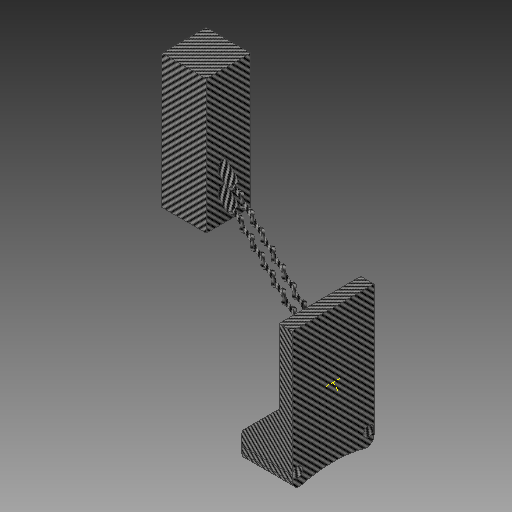
# Autodesk Inventor part: lower clamp
Saved by Autodesk Inventor 2018 (Build 220112000, 112)
## iProperties
Created: 2021-03-10
Part Number: lower clamp
Material: CFRP
Document SubType Name: Modeling
Designer: Hp
Density: 1.43 g/cm^3
Appearance: Carbon Fiber
Author: Hp
Autodesk Inventor part; units mm, degrees
sketch "Sketch1" plane through (0, 0, 0) normal (0, 1, 0) x (-1, 0, 0)
  line L0 (0, 0) -> (34, 0)
  line L1 (34, 0) -> (34, -55)
  line L2 (34, -55) -> (0, -55)
  line L3 (0, -55) -> (0, 0)
  dimension "d0" = 34
  dimension "d1" = 55
  dimension "d2" = 90
  dimension "d3" = 34
  dimension "d4" = 90
  constraints: 8 end point, 2 perpendicular, 1 horizontal
  measures "d0" distance of L0.start L0.end
  measures "d1" distance of L0.end L1.end
  measures "d2" angle of L0 L1
  measures "d3" distance of L1.end L2.end
  measures "d4" angle of L1 L2
extrude "Extrusion1" add sketch "Sketch1" along normal blind 9
sketch "Sketch2" plane through (0, 0, 0) normal (1, 0, 0) x (0, 0, -1)
  line L0 (55, 0) -> (0, 0) projected
  arc A0 (7, 0) -> (0, 0) centre (3.5, 0) ccw
  arc A1 (55, 0) -> (48, 0) centre (51.5, 0) ccw
  dimension "d7" = 7
  dimension "d8" = 7
  constraints: 4 point on circle, 4 point on line, 2 centre point, 2 end point
  measures "d7" diameter of A0
  measures "d8" diameter of A1
extrude "Extrusion2" cut sketch "Sketch2" against normal blind 1000
sketch "Sketch3" plane through (-34, 9, 0) normal (0, 0, 1) x (1, 0, 0)
  line L0 (0, 0) -> (34, 0) projected
  line L1 (34, 0) -> (34, 50)
  line L2 (0, 0) -> (25, 25)
  line L3 (0, 0) -> (50.7113, 0) construction
  line L4 (25, 25) -> (25, 50) construction
  line L5 (25, 25) -> (25, 50)
  line L6 (34, 50) -> (25, 50)
  point P0 (34, -9)
  dimension "d11" = 50
  dimension "d12" = 45
  dimension "d13" = 9
  constraints: 12 end point, 2 vertical, 1 collinear, 1 horizontal, 1 perpendicular
  measures "d11" distance of L0.end L1.end
  measures "d12" angle of L3 L2
  measures "d13" distance of L1.end L4.end
extrude "Extrusion3" add sketch "Sketch3" against normal blind 55
sketch "Sketch4" plane through (0, 0, 0) normal (0, -1, 0) x (1, 0, 0)
  line L0 (-34, -55) -> (-9, -55) projected
  line L1 (-9, 0) -> (-34, 0) projected
  circle A0 centre (-17, -27.5) radius 3.5
  point P0 (0, 0)
  dimension "d16" = 7
  constraints: 1 centre point
  measures "d16" diameter of A0
extrude "Extrusion4" add sketch "Sketch4" against normal blind 30 and the other way blind 10
sketch "Sketch5" plane through (-9, 59, 0) normal (0, 1, 0) x (1, 0, 0)
  line L0 (0, 0) -> (0, 55) projected
  line L1 (0, 55) -> (9, 55) projected
  line L2 (0, 0) -> (9, 0)
  line L3 (9, 0) -> (9, 55)
  line L4 (9, 55) -> (0, 55)
  line L5 (0, 55) -> (0, 0)
  constraints: 8 end point, 2 parallel, 1 horizontal, 1 perpendicular
extrude "Extrusion5" add sketch "Sketch5" along normal blind 5
sketch "Sketch7" plane through (0, 0, -7) normal (1, 0, 0) x (0, 0, -1)
  circle A0 centre (20.5, 44) radius 3.5 projected
  circle A1 centre (20.5, 44) radius 3.5
  circle A2 centre (20.5, 54) radius 3.5 projected
  circle A3 centre (20.5, 54) radius 3.5
  point P0 (-7, 0)
  constraints: 2 centre point, 2 coincident
extrude "Extrusion7" add sketch "Sketch7" against normal blind 9
sketch "Sketch15" plane through (-9, 64, 0) normal (0, 1, 0) x (1, 0, 0)
  line L0 (-25, 55) -> (9, 55) projected
  line L1 (0, 0) -> (9, 0)
  line L2 (9, 0) -> (9, 55)
  line L3 (9, 55) -> (0, 55)
  line L4 (0, 55) -> (0, 0)
  constraints: 8 end point, 2 parallel, 1 horizontal, 1 perpendicular
extrude "Extrusion9" add sketch "Sketch15" along normal blind 20
ref_plane "Work Plane4" through (-9, 84, -55) normal (-0.7071068, 0.7071068, 0) x (0, 0, 1)
sketch "Sketch17" plane through (-9, 84, -55) normal (-0.7071068, 0.7071068, 0) x (0, 0, 1)
  line L0 (0, 0) -> (55, 0) construction
  line L1 (27.5, 0) -> (27.5, -14.414) construction
  circle A0 centre (27.5, -14.414) radius 3.5 construction
  circle A1 centre (27.5, -14.414) radius 3.5
  line L2 (27.5, -14.414) -> (27.5, -24.414) construction
  circle A2 centre (27.5, -24.414) radius 3.5 construction
  circle A3 centre (27.5, -24.414) radius 3.5
  point P0 (55, -53.033)
  dimension "d49" = 14.414
  dimension "d50" = 7
  dimension "d51" = 10
  dimension "d52" = 7
  dimension "d53" = 7
  constraints: 4 centre point, 4 coincident, 4 end point, 1 concentric, 1 midpoint, 1 point on line, 1 vertical
  measures "d49" distance of L1.start L1.end
  measures "d50" diameter of A0
  measures "d51" distance of L2.start L2.end
  measures "d52" diameter of A2
  measures "d53" diameter of A3
extrude "Extrusion11" cut sketch "Sketch17" against normal blind 200
sketch "Sketch18" plane through (0, 40.4734, -27.5) normal (0.7071068, 0.7071068, 0) x (0, 0, -1)
  point P0 (0, 0)
sketch "Sketch19" plane through (0, 40.4734, -27.5) normal (-0.7071068, 0.7071068, 0) x (0.7071068, 0.7071068, 0)
  circle A0 centre (0, 0) radius 3.5
  circle A1 centre (0, 0) radius 2.5
  dimension "d68" = 5
  constraints: 2 centre point, 2 coincident
  measures "d68" diameter of A1
extrude "Extrusion12" add sketch "Sketch19" along normal blind 20 and the other way blind 10
sketch "Sketch21" plane through (0, 40.4734, -27.5) normal (-0.7071068, 0.7071068, 0) x (0.7071068, 0.7071068, 0)
  circle A0 centre (0, 0) radius 2.5
  constraints: 1 centre point, 1 coincident
extrude "Extrusion13" add sketch "Sketch21" along normal blind 18 and the other way blind 10
sketch "Sketch23" plane through (-12.7279, 53.2013, -27.5) normal (-0.7071068, 0.7071068, 0) x (-0.7071068, -0.7071068, 0)
  circle A0 centre (-1.5, 0) radius 1
  point P0 (28.619, 27.5)
  constraints: 1 centre point
coil "Coil1" sketch "Sketch23" operation add axis through (7.0711, 33.4023, -27.5) along (-0.7071068, 0.7071068, 0) pitch 10 turns 8 hand right
sketch "Sketch24" plane through (0, 54.6155, -27.5) normal (-0.7071068, 0.7071068, 0) x (-0.7071068, -0.7071068, 0)
  circle A0 centre (0, 0) radius 3.5
  circle A1 centre (0, 0) radius 2.5
  dimension "d91" = 5
  constraints: 2 centre point, 2 coincident
  measures "d91" diameter of A1
extrude "Extrusion14" add sketch "Sketch24" along normal blind 20 and the other way blind 10
sketch "Sketch25" plane through (0, 54.6155, -27.5) normal (0, 0, 1) x (-0.7071068, 0.7071068, 0)
  point P0 (0, 0)
sketch "Sketch26" plane through (0, 54.6155, -27.5) normal (-0.7071068, 0.7071068, 0) x (-0.7071068, -0.7071068, 0)
  circle A0 centre (0, 0) radius 2.5
  constraints: 1 centre point, 1 coincident
extrude "Extrusion15" add sketch "Sketch26" along normal blind 18 and the other way blind 10
sketch "Sketch27" plane through (-12.7279, 67.3434, -27.5) normal (-0.7071068, 0.7071068, 0) x (-0.7071068, -0.7071068, 0)
  point P0 (38.619, 27.5)
sketch "Sketch28" plane through (-12.7279, 67.3434, -27.5) normal (-0.7071068, 0.7071068, 0) x (-0.7071068, -0.7071068, 0)
  circle A0 centre (-1.5, 0) radius 1
  point P0 (38.619, 27.5)
  dimension "d96" = 2
  constraints: 1 centre point
  measures "d96" diameter of A0
coil "Coil2" sketch "Sketch28" operation add axis through (7.0711, 47.5445, -27.5) along (-0.7071068, 0.7071068, 0) pitch 10 turns 8 hand right
ref_plane "Work Plane5" through (-70.7107, 111.1841, -27.5) normal (-0.7071068, 0.7071068, 0) x (-0.7071068, -0.7071068, 0)
sketch "Sketch29" plane through (-70.7107, 111.1841, -27.5) normal (-0.7071068, 0.7071068, 0) x (-0.7071068, -0.7071068, 0)
  circle A0 centre (0, 0) radius 2.5
  circle A1 centre (0, 0) radius 3.5
  point P0 (28.619, 27.5)
  point P1 (-0.7725, -2.3776)
  constraints: 2 coincident, 1 centre point, 3 other
extrude "Extrusion16" add sketch "Sketch29" along normal blind 50 and the other way blind 5 contours A0 | A1
ref_plane "Work Plane6" through (-70.7107, 125.3262, -27.5) normal (-0.7071068, 0.7071068, 0) x (-0.7071068, -0.7071068, 0)
sketch "Sketch30" plane through (-70.7107, 125.3262, -27.5) normal (-0.7071068, 0.7071068, 0) x (-0.7071068, -0.7071068, 0)
  circle A0 centre (0, 0) radius 3.5 projected
  circle A1 centre (0, 0) radius 3.5
  point P0 (38.619, 27.5)
  constraints: 1 centre point, 1 coincident
extrude "Extrusion17" add sketch "Sketch30" along normal blind 50 and the other way blind 5
ref_plane "Work Plane7" through (-89, 34, -55) normal (-1, 0, 0) x (0, 0, 1)
sketch "Sketch31" plane through (-89, 34, -55) normal (-1, 0, 0) x (0, 0, 1)
  line L0 (9, 62.2361) -> (39, 62.2361)
  line L1 (39, 62.2361) -> (39, 152.2361)
  line L2 (39, 152.2361) -> (9, 152.2361)
  line L3 (9, 152.2361) -> (9, 62.2361)
  line L4 (24, 87.7907) -> (24, 126.6815) projected
  line L5 (9, 62.2361) -> (39, 152.2361) construction
  line L6 (39, 62.2361) -> (9, 152.2361) construction
  point P0 (55, -34)
  point P1 (24, 107.2361)
  dimension "d122" = 30
  dimension "d123" = 90
  constraints: 12 end point, 3 midpoint, 2 parallel, 1 horizontal, 1 perpendicular
  measures "d122" distance of L2.end L1.end
  measures "d123" distance of L1.end L0.end
extrude "Extrusion18" add sketch "Sketch31" against normal blind 15 and the other way blind 15
sketch "Sketch32" plane through (0, 0, 0) normal (0, -1, 0) x (1, 0, 0)
  line L0 (-34, -55) -> (0, -55)
  line L1 (0, -55) -> (0, 0)
  line L2 (0, 0) -> (-34, 0)
  line L3 (-34, 0) -> (-34, -55)
  circle A0 centre (-17, -27.5) radius 3.5 projected
  line L4 (-34, -55) -> (0, 0) construction
  line L5 (0, -55) -> (-34, 0) construction
  constraints: 12 end point, 2 midpoint, 2 parallel, 1 horizontal, 1 perpendicular
extrude "Extrusion19" add sketch "Sketch32" along normal blind 9
mirror "Mirror1" about plane through (-17, 0, -27.5) normal (0, 1, 0) of "Extrusion2"
sketch "Sketch33" plane through (0, 84, 0) normal (1, 0, 0) x (0, 0, -1)
  line L0 (55, -93) -> (0, -93) projected
  line L1 (55, 0) -> (0, 0)
  line L2 (0, 0) -> (0, -93)
  line L3 (0, -93) -> (55, -93)
  line L4 (55, -93) -> (55, 0)
  point P0 (0, -84)
  constraints: 8 end point, 2 parallel, 1 horizontal, 1 perpendicular
extrude "Extrusion20" cut sketch "Sketch33" along normal blind 900
sketch "Sketch34" plane through (-104, 34, -55) normal (-1, 0, 0) x (0, 0, 1)
  line L0 (39, 152.2361) -> (9, 152.2361) projected
  line L1 (39, 62.2361) -> (39, 152.2361) projected
  line L2 (9, 152.2361) -> (39, 152.2361)
  line L3 (39, 152.2361) -> (39, 62.2361)
  line L4 (39, 62.2361) -> (9, 62.2361)
  line L5 (9, 62.2361) -> (9, 152.2361)
  point P0 (55, -34)
  constraints: 8 end point, 2 parallel, 1 horizontal, 1 perpendicular
extrude "Extrusion21" cut sketch "Sketch34" along normal blind 900
sketch "Sketch36" plane through (-67.1751, 121.7907, -27.5) normal (0.7071068, -0.7071068, 0) x (-0.7071068, -0.7071068, 0)
  circle A0 centre (0, 0) radius 1
  point P0 (38.619, -27.5)
  dimension "d142" = 2
  constraints: 1 centre point
  measures "d142" diameter of A0
extrude "Extrusion22" add sketch "Sketch36" along normal blind 90
sketch "Sketch37" plane through (-67.1751, 107.6485, -27.5) normal (0.7071068, -0.7071068, 0) x (-0.7071068, -0.7071068, 0)
  circle A0 centre (0, 0) radius 1
  point P0 (28.619, -27.5)
  dimension "d145" = 2
  constraints: 1 centre point
  measures "d145" diameter of A0
extrude "Extrusion23" add sketch "Sketch37" along normal blind 90
fillet "Fillet1" radius 5 1 edges at (-34, 9, -27.5)
fillet "Fillet2" radius 5 2 edges at (-17, -9, -55) (-17, -9, 0)
sketch "Sketch39" plane through (-34, 0, -3.5) normal (-1, 0, 0) x (0, 0, 1)
  line L0 (-1.5, -9) -> (-46.5, -9) projected
  arc A0 (-51.5, -4) -> (-46.5, -9) centre (-46.5, -4) ccw projected
  arc A1 (-1.5, -9) -> (-46.5, -9) centre (-24, -87.6764) ccw
  line L1 (-1.5, -9) -> (-46.5, -9)
  point P0 (3.5, 0)
  constraints: 2 end point, 2 point on circle, 1 centre point, 1 collinear
extrude "Extrusion24" cut sketch "Sketch39" against normal blind 90
ref_plane "Work Plane10" through (-10.4142, 35.4142, -55) normal (-0.7071068, 0.7071068, 0) x (-0.7071068, -0.7071068, 0)
sketch "Sketch44" plane through (-10.4142, 35.4142, -55) normal (-0.7071068, 0.7071068, 0) x (-0.7071068, -0.7071068, 0)
  ellipse E0 centre (11.3137, 27.5) end of major axis (16.2635, 27.5) minor radius 3.5 projected
  circle A0 centre (11.3137, 27.5) radius 5
  point P0 (17.6777, 55)
  dimension "d163" = 10
  constraints: 1 centre point, 1 coincident, 1 other
  measures "d163" diameter of A0
extrude "Extrusion27" add sketch "Sketch44" along normal blind 5 and the other way blind 2.5 contours E0 | A0
fillet "Fillet4" radius 3 1 edges at (-18.4142, 34.4853, -27.5)
sketch "Sketch45" plane through (-104, 96.2361, -46) normal (0, -1, 0) x (1, 0, 0)
  line L0 (2, 2) -> (28, 2)
  line L1 (28, 2) -> (28, 28)
  line L2 (28, 28) -> (2, 28)
  line L3 (2, 28) -> (2, 2)
  point P0 (104, 46)
  dimension "d169" = 26
  dimension "d170" = 26
  constraints: 8 end point, 2 parallel, 1 horizontal, 1 perpendicular
  measures "d169" distance of L2.end L1.end
  measures "d170" distance of L1.end L0.end
extrude "Extrusion28" cut sketch "Sketch45" against normal blind 2
body "Solid1"
